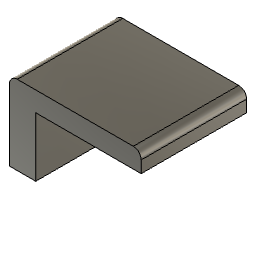
Laptop Hold Vertical v2 (Autodesk Fusion 360 design; units mm, degrees)
Autodesk Fusion 360 part; units mm, degrees
note: some values were not read from the file. Chosen so that the rebuilt part matches the saved one: a direction.
sketch "Sketch1" plane through (0, 0, 0) normal (0, 1, 0) x (1, 0, 0)
  line L0 (0, 0) -> (0, -30)
  line L1 (0, -30) -> (50, -30)
  line L2 (50, -30) -> (50, -22.5)
  line L3 (50, -22.5) -> (10, -22.5)
  line L4 (10, -22.5) -> (10, 0)
  line L5 (10, 0) -> (0, 0)
  dimension "d1" = 10
  dimension "d2" = 30
  dimension "d3" = 50
  dimension "d9" = 7.5
  constraint coincident L0.start L5.end
  constraint vertical L0
  constraint perpendicular L0 L1
  constraint perpendicular L1 L2
  constraint perpendicular L2 L3
  constraint perpendicular L3 L4
  constraint perpendicular L0 L5
  measures "d1" distance of L4.end L0.start
  measures "d2" distance of L0.start L0.end
  measures "d3" distance of L0.end L1.end
  measures "d9" distance of L1.end L2.end
extrude "Extrude1" add sketch "Sketch1" along normal blind 40
sketch "Sketch2" plane through (10, 0, 0) normal (1, 0, 0) x (0, 1, 0)
  line L0 (0, 22.5) -> (0, 0)
  line L1 (0, 0) -> (40, 0)
  line L2 (40, 0) -> (40, 22.5)
  line L3 (40, 22.5) -> (0, 22.5)
  line L4 (23.25, 15) -> (23.25, 7.5)
  line L5 (16.75, 7.5) -> (16.75, 15)
  arc A0 (23.25, 15) -> (16.75, 15) centre (20, 15) ccw
  arc A1 (16.75, 7.5) -> (23.25, 7.5) centre (20, 7.5) ccw
  line L6 (0, 0) -> (40, 22.5) construction
  line L7 (20, 15) -> (20, 7.5) construction
  dimension "d6" = 6.5
  dimension "d7" = 7.5
  constraint vertical L4
  constraint vertical L5
  constraint tangent L5 A0
  constraint tangent L5 A1
  constraint tangent L4 A1
  constraint tangent L4 A0
  constraint coincident L0.end L1.start
  constraint coincident L2.end L3.start
  constraint coincident A0.centre L7.start
  constraint coincident A1.centre L7.end
  constraint midpoint L6 L7
  measures "d6" distance of L4 L5
  measures "d7" distance of L4.start L4.end
extrude "Extrude2" cut sketch "Sketch2" against normal through all contours L4 L5 A0 A1
fillet "Fillet1" radius 3 2 edges at (0, 20, 30) (50, 20, 30)
